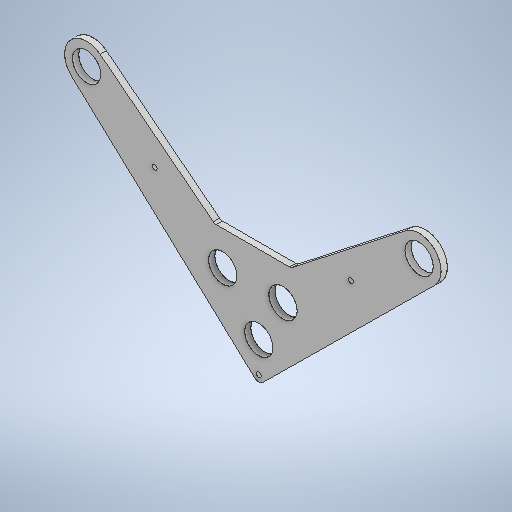
# Autodesk Inventor part: Gearbox #2 Top Plate
Saved by Autodesk Inventor 2025.1 (Build 291241020, 241B)
## iProperties
Created: 2024-09-29
Part Number: Gearbox #2 Top Plate
Material: Generic
Document SubType Name: Modeling
Designer: xmand
Density: 1 g/cm^3
Appearance: Default
Author: xmand
Autodesk Inventor part; units mm, degrees
ref_plane "YZ Plane" through (0, 0, 0) normal (1, 0, 0) x (0, 1, 0)
ref_plane "XZ Plane" through (0, 0, 0) normal (0, 1, 0) x (-1, 0, 0)
ref_plane "XY Plane" through (0, 0, 0) normal (0, 0, 1) x (1, 0, 0)
sketch "Sketch1" plane through (60.3372, -82.808, 0) normal (0, 0, 1) x (1, 0, 0)
  circle A0 centre (0, 0) radius 20.32 construction
  circle A1 centre (0, 0) radius 22.86 construction
  circle A2 centre (24.5471, 44.4756) radius 30.48 construction
  circle A3 centre (-36.4129, 44.4756) radius 30.48 construction
  circle A4 centre (-36.4129, 44.4756) radius 33.02 construction
  line L0 (-15.4952, 18.9262) -> (-14.4815, 17.688)
  circle A5 centre (24.5471, 44.4756) radius 33.02 construction
  circle A6 centre (24.5471, 44.4756) radius 14.2875
  circle A7 centre (-36.4129, 44.4756) radius 14.2875
  circle A8 centre (0, 0) radius 14.2875
  circle A9 centre (24.5471, 44.4756) radius 19.1008 construction
  circle A10 centre (24.5471, 44.4756) radius 21.0058 construction
  circle A11 centre (-36.4129, 44.4756) radius 19.1008 construction
  circle A12 centre (-36.4129, 44.4756) radius 21.0058 construction
  line L1 (-36.4129, 44.4756) -> (-174.0993, 152.048) construction
  line L2 (24.5471, 44.4756) -> (162.2336, 152.048) construction
  circle A13 centre (-174.0993, 152.048) radius 14.2875
  circle A14 centre (162.2336, 152.048) radius 14.2875
  circle A15 centre (-174.0993, 152.048) radius 22.225 construction
  circle A16 centre (162.2336, 152.048) radius 22.225 construction
  line L3 (-160.4162, 169.5616) -> (-45.921, 80.1081)
  line L4 (-42.9811, 79.0958) -> (31.1154, 79.0958)
  arc A17 (31.1154, 79.0958) -> (34.0553, 80.1081) centre (31.1154, 83.871) ccw
  arc A18 (-45.921, 80.1081) -> (-42.9811, 79.0958) centre (-42.9811, 83.871) ccw
  line L5 (34.0553, 80.1081) -> (148.5505, 169.5616)
  line L6 (-36.4129, 79.0958) -> (-36.4129, 77.4956) construction
  arc A19 (177.8656, 136.2496) -> (148.5505, 169.5616) centre (162.2336, 152.048) ccw
  arc A20 (-160.4162, 169.5616) -> (-189.2001, 135.7411) centre (-174.0993, 152.048) ccw
  circle A21 centre (-105.2561, 98.2618) radius 2.4892
  circle A22 centre (0, -30.8102) radius 6.35 construction
  circle A23 centre (0, -30.8102) radius 2.4892
  line L7 (0, -22.86) -> (0, -24.4602)
  line L8 (-189.2001, 135.7411) -> (-4.3145, -35.4693)
  line L9 (177.8656, 136.2496) -> (4.4663, -35.324)
  arc A24 (-4.3145, -35.4693) -> (4.4663, -35.324) centre (0, -30.8102) ccw
  circle A25 centre (-105.2561, 98.2618) radius 6.35 construction
  circle A26 centre (93.3904, 98.2618) radius 6.35 construction
  circle A27 centre (93.3904, 98.2618) radius 2.4892
  circle A28 centre (-174.0993, 152.048) radius 50.8 construction
  circle A29 centre (162.2336, 152.048) radius 50.8 construction
  line L10 (-333.708, 192.5945) -> (-312.3217, 152.048) construction
  dimension "d25" = 40.64
  dimension "d24" = 2.54
  dimension "d23" = 60.96
  dimension "d22" = 2.54
  dimension "d21" = 1.6002
  dimension "d20" = 28.575
  dimension "d19" = 38.2016
  dimension "d18" = 42.0116
  dimension "d17" = 174.7266
  dimension "d16" = 104
  dimension "d15" = 28.575
  dimension "d14" = 44.45
  dimension "d13" = 44.45
  dimension "d12" = 4.7752
  dimension "d11" = 1.6002
  dimension "d9" = 4.9784
  dimension "d8" = 12.7
  dimension "d7" = 4.9784
  dimension "d6" = 1.6002
  dimension "d5" = 12.7
  dimension "d3" = 12.7
  dimension "d2" = 4.9784
  dimension "d10" = 87.3633
  dimension "d4" = 87.3633
  dimension "d0" = 101.6
  dimension "d1" = 101.6
  constraints: 30 centre point, 22 coincident, 22 end point, 21 point on circle, 16 tangent, 9 equal radius, 6 point on line, 2 horizontal alignment, 2 midpoint, 2 parallel, 2 vertical, 1 equal length, 1 horizontal
  measures "d25" diameter of A0
  measures "d24" radial gap between concentric circles of A1 A0
  measures "d23" diameter of A2
  measures "d22" radial gap between concentric circles of A3 A4
  measures "d21" distance of L0.start L0.end
  measures "d20" diameter of A6
  measures "d19" diameter of A9
  measures "d18" diameter of A10
  measures "d17" distance of L1.start L1.end
  measures "d16" angle of L2 L1
  measures "d15" diameter of A13
  measures "d14" diameter of A15
  measures "d13" diameter of A16
  measures "d12" radius of A18
  measures "d11" distance of L6.start L6.end
  measures "d9" diameter of A21
  measures "d8" diameter of A22
  measures "d7" diameter of A23
  measures "d6" distance of L7.start L7.end
  measures "d5" diameter of A25
  measures "d3" diameter of A26
  measures "d2" diameter of A27
  measures "d10" distance of A3.centre A21.centre
  measures "d4" distance of A26.centre A2.centre
  measures "d0" diameter of A29
  measures "d1" diameter of A28
extrude "Extrusion1" add sketch "Sketch1" along normal mid plane 6.35
body "Solid1"
